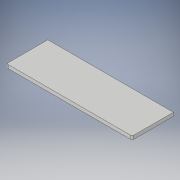
# Autodesk Inventor part: key board 1
Saved by Autodesk Inventor 2017 (Build 210142000, 142)
## iProperties
Created: 2018-03-14
Part Number: key board 1
Material: Generic
Document SubType Name: Modeling
Designer: braxtonwright
Density: 1 g/cm^3
Appearance: Default
Author: braxtonwright
Autodesk Inventor part; units mm, degrees
ref_plane "YZ Plane" through (0, 0, 0) normal (1, 0, 0) x (0, 1, 0)
ref_plane "XZ Plane" through (0, 0, 0) normal (0, 1, 0) x (-1, 0, 0)
ref_plane "XY Plane" through (0, 0, 0) normal (0, 0, 1) x (1, 0, 0)
sketch "Sketch1" plane through (0, 0, 0) normal (0, 1, 0) x (-1, 0, 0)
  line L0 (-0.5292, 0) -> (-36.5125, 0)
  line L1 (-37.0417, -0.5292) -> (-37.0417, -12.1708)
  line L2 (-37.0417, -12.1708) -> (0, -12.1708)
  line L3 (0, -12.1708) -> (0, -0.5292)
  arc A0 (0, -0.5292) -> (-0.5292, 0) centre (-0.5292, -0.5292) ccw
  line L4 (-18.5208, -12.969) -> (-18.5208, 2.8326) construction
  arc A1 (-36.5125, 0) -> (-37.0417, -0.5292) centre (-36.5125, -0.5292) ccw
  point P0 (0, 0)
  dimension "d4" = 1.0583
  dimension "d5" = 12.1708
  dimension "d6" = 37.0417
  constraints: 10 end point, 4 point on circle, 3 perpendicular, 2 centre point, 1 horizontal, 1 symmetric about line, 1 vertical, 1 other
  measures "d4" diameter of A0
  measures "d5" distance between parallel lines of L0 L2
  measures "d6" distance between parallel lines of L1 L3
extrude "main key board" add sketch "Sketch1" along normal blind 1.0583
body "Solid1"
